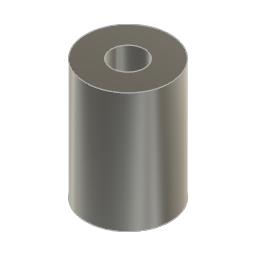
shaft size v4 (Autodesk Fusion 360 design; units mm, degrees)
Autodesk Fusion 360 part; units mm, degrees
sketch "Sketch1" plane through (0, 0, 0) normal (0, 0, 1) x (1, 0, 0)
  circle A0 centre (0, 0) radius 3.5
  circle A1 centre (0, 0) radius 1.375
  dimension "d1" = 2.75
  dimension "d12" = 7
  constraint coincident A0.centre A1.centre
  measures "d1" diameter of A1
  measures "d12" diameter of A0
extrude "Extrude1" add sketch "Sketch1" along normal blind 10
